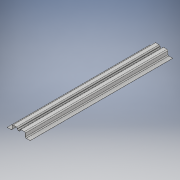
# Autodesk Inventor part: AAD0001145625
Saved by Autodesk Inventor 2017 (Build 210142000, 142)
## iProperties
Created: 2019-04-10
Part Number: AAD0001145625
Material: Generic
Document SubType Name: Modeling
Designer: Phs
Density: 1 g/cm^3
Appearance: Default
Author: Phs
Autodesk Inventor part; units mm, degrees
ref_plane "YZ Plane" through (0, 0, 0) normal (1, 0, 0) x (0, 1, 0)
ref_plane "XZ Plane" through (0, 0, 0) normal (0, 1, 0) x (-1, 0, 0)
ref_plane "XY Plane" through (0, 0, 0) normal (0, 0, 1) x (1, 0, 0)
sketch "Sketch1" plane through (0, 0, 0) normal (0, 0, 1) x (1, 0, 0)
  line L0 (0, 14.3) -> (0, 15.1)
  line L1 (-6.95, 19.1) -> (-6.95, 20.3)
  line L2 (0, 14.3) -> (-2.15, 14.3)
  line L3 (-32.2, 4.8) -> (-32.2, 20.3)
  line L4 (-10.95, 24.3) -> (-28.2, 24.3)
  line L5 (-37, 0) -> (-56.95, 0)
  arc A0 (-6.95, 19.1) -> (-2.15, 14.3) centre (-2.15, 19.1) ccw
  arc A1 (-37, 0) -> (-32.2, 4.8) centre (-37, 4.8) ccw
  arc A2 (-28.2, 24.3) -> (-32.2, 20.3) centre (-28.2, 20.3) ccw
  arc A3 (-6.95, 20.3) -> (-10.95, 24.3) centre (-10.95, 20.3) ccw
  line L6 (-56.95, 0.8) -> (-37, 0.8)
  arc A4 (-37, 0.8) -> (-33, 4.8) centre (-37, 4.8) ccw
  line L7 (-33, 4.8) -> (-33, 20.3)
  arc A5 (-28.2, 25.1) -> (-33, 20.3) centre (-28.2, 20.3) ccw
  line L8 (-28.2, 25.1) -> (-10.95, 25.1)
  arc A6 (-6.15, 20.3) -> (-10.95, 25.1) centre (-10.95, 20.3) ccw
  line L9 (-6.15, 20.3) -> (-6.15, 19.1)
  arc A7 (-6.15, 19.1) -> (-2.15, 15.1) centre (-2.15, 19.1) ccw
  line L10 (-2.15, 15.1) -> (0, 15.1)
  line L11 (-56.95, 0) -> (-56.95, 0.8)
  point P0 (0, 0)
  dimension "d0" = 6.95
  dimension "d1" = 25.25
  dimension "d2" = 14.3
  dimension "d3" = 10
  dimension "d4" = 4.8
  dimension "d5" = 4
  dimension "d6" = 19.95
  dimension "d7" = 0.8
  constraints: 24 end point, 16 point on circle, 8 centre point, 8 tangent, 5 parallel, 2 equal radius, 2 horizontal, 2 vertical, 7 other
  measures "d0" distance between parallel lines of L0 L1
  measures "d1" distance between parallel lines of L1 L3
  measures "d2" distance from line of L2 point (0, 0)
  measures "d3" distance between parallel lines of L2 L4
  measures "d4" radius of A0
  measures "d5" radius of A2
  measures "d6" distance of L5.start L5.end
  measures "d7" distance between parallel lines of L4 L8
extrude "Extrusion1" add sketch "Sketch1" along normal mid plane 707
mirror "Mirror1" about plane through (0, 0, 0) normal (1, 0, 0) of "Extrusion1"
body "Solid1"
